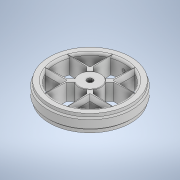
# Autodesk Inventor part: custom_wheel_v6
Saved by Autodesk Inventor 2022 (Build 260153000, 153)
## iProperties
Created: 2023-01-27
Part Number: custom_wheel_v6
Material: Generic
Document SubType Name: Modeling
Designer: user
Density: 1 g/cm^3
Appearance: Default
Author: user
Autodesk Inventor part; units mm, degrees
ref_plane "YZ Plane" through (0, 0, 0) normal (1, 0, 0) x (0, 1, 0)
ref_plane "XZ Plane" through (0, 0, 0) normal (0, 1, 0) x (-1, 0, 0)
ref_plane "XY Plane" through (0, 0, 0) normal (0, 0, 1) x (1, 0, 0)
sketch "Sketch1" plane through (0, 0, 0) normal (0, 1, 0) x (-1, 0, 0)
  circle A0 centre (0, 0) radius 37.5
  circle A1 centre (0, 0) radius 30
  circle A2 centre (0, 0) radius 10
  circle A3 centre (0, 0) radius 2.6
  dimension "d0" = 75
  dimension "d1" = 60
  dimension "d2" = 20
  dimension "d3" = 5.2
  constraints: 4 centre point, 4 coincident
  measures "d0" diameter of A0
  measures "d1" diameter of A1
  measures "d2" diameter of A2
  measures "d3" diameter of A3
extrude "Extrusion1" add sketch "Sketch1" along normal blind 15
sketch "Sketch2" plane through (0, 15, 0) normal (0, 1, 0) x (1, 0, 0)
  line L0 (0, 2.35) -> (1.1124, 2.35)
  circle A0 centre (0, 0) radius 2.6 projected
  line L1 (0, 2.35) -> (-1.1124, 2.35)
  constraints: 4 end point, 2 horizontal, 2 point on circle
extrude "Extrusion2" add sketch "Sketch2" against normal blind 15 contours L1 A0 L0 picked at (-0.5608, 2.4122)
sketch "Sketch3" plane through (-1.1124, 15, -2.35) normal (0, 0, 1) x (1, 0, 0)
  line L0 (2.2249, 0) -> (2.2249, -15) projected
  line L1 (2.2249, 0) -> (2.2249, -15)
  line L2 (11.1124, -15) -> (-8.8876, -15) projected
  line L3 (-1.4876, 0) -> (-1.4876, -15) projected
  line L4 (-1.4876, 0) -> (-1.4876, -15)
  line L5 (0, 0) -> (2.2249, 0) projected
  line L6 (1.1124, 0) -> (1.1124, -15)
  line L7 (-1.4876, -15) -> (3.7124, -15) projected
  circle A0 centre (1.1124, -7.5) radius 1.4
  point P0 (0, -15)
  point P1 (1.1124, -6.1)
  point P2 (1.1124, -8.9)
  point P3 (2.2249, -6.65)
  point P4 (2.2249, -8.35)
  dimension "d8" = 2.8
  constraints: 6 end point, 3 point on line, 2 midpoint, 1 centre point, 1 perpendicular, 1 vertical
  measures "d8" diameter of A0
extrude "Extrusion3" cut sketch "Sketch3" against normal blind 85 contours A0 L0 | L0 A0 L6 | L6 A0
sketch "Sketch5" plane through (0, 15, 0) normal (0, 1, 0) x (1, 0, 0)
  circle A0 centre (0, 0) radius 36.25
  arc A1 (-1.1124, 2.35) -> (1.1124, 2.35) centre (0, 0) ccw projected
  circle A2 centre (0, 0) radius 37.5
  dimension "d17" = 72.5
  constraints: 2 centre point, 2 coincident
  measures "d17" diameter of A0
extrude "Extrusion5" cut sketch "Sketch5" against normal blind 2.75
sketch "Sketch6" plane through (0, 0, 0) normal (0, -1, 0) x (1, 0, 0)
  circle A0 centre (0, 0) radius 37.5
  circle A1 centre (0, 0) radius 36.25
  dimension "d20" = 72.5
  constraints: 2 centre point, 2 coincident
  measures "d20" diameter of A1
extrude "Extrusion6" cut sketch "Sketch6" against normal blind 2.75
chamfer "Chamfer1" distance 1.25 angle 45 2 edges at (37.5, 12.25, 0) (37.5, 2.75, 0)
fillet "Fillet1" radius 0.4125 2 edges at (10, 0, 0) (10, 15, 0)
sketch "Sketch8" plane through (0, 15, 0) normal (0, 1, 0) x (1, 0, 0)
  line L0 (0, 0) -> (7.0711, 7.0711)
  circle A0 centre (0, 0) radius 10 projected
  line L1 (0, 0) -> (10, 0) construction
  line L2 (6.1527, 6.1527) -> (4.7385, 7.5669)
  line L3 (4.7385, 7.5669) -> (7.5669, 4.7385)
  line L4 (7.5669, 4.7385) -> (14.638, 11.8096)
  line L5 (14.638, 11.8096) -> (11.8096, 14.638)
  line L6 (11.8096, 14.638) -> (4.7385, 7.5669)
  line L7 (13.2238, 13.2238) -> (13.2238, 29.2831)
  line L8 (13.2238, 29.2831) -> (10, 30)
  line L9 (10, 30) -> (8.9811, 11.8096)
  line L10 (13.2238, 13.2238) -> (6.1527, 6.1527)
  line L11 (13.2238, 13.2238) -> (29.2831, 13.2238)
  line L12 (29.2831, 13.2238) -> (30, 10)
  line L13 (30, 10) -> (11.8096, 8.9811)
  line L14 (-13.2238, 13.2238) -> (-29.2831, 13.2238)
  line L15 (-30, 10) -> (-11.8096, 8.9811)
  line L16 (-29.2831, 13.2238) -> (-30, 10)
  line L17 (-4.7385, 7.5669) -> (-11.8096, 14.638)
  line L18 (-6.1527, 6.1527) -> (-7.5669, 4.7385)
  line L19 (-7.5669, 4.7385) -> (-4.7385, 7.5669)
  line L20 (-14.638, 11.8096) -> (-7.5669, 4.7385)
  line L21 (-13.2238, 13.2238) -> (-13.2238, 29.2831)
  line L22 (-10, 30) -> (-8.9811, 11.8096)
  line L23 (-13.2238, 29.2831) -> (-10, 30)
  line L24 (-11.8096, 14.638) -> (-14.638, 11.8096)
  line L25 (-13.2238, -13.2238) -> (-13.2238, -29.2831)
  line L26 (-10, -30) -> (-8.9811, -11.8096)
  line L27 (-13.2238, -29.2831) -> (-10, -30)
  line L28 (-7.5669, -4.7385) -> (-14.638, -11.8096)
  line L29 (-6.1527, -6.1527) -> (-4.7385, -7.5669)
  line L30 (-4.7385, -7.5669) -> (-7.5669, -4.7385)
  line L31 (-11.8096, -14.638) -> (-4.7385, -7.5669)
  line L32 (-13.2238, -13.2238) -> (-29.2831, -13.2238)
  line L33 (-30, -10) -> (-11.8096, -8.9811)
  line L34 (-29.2831, -13.2238) -> (-30, -10)
  line L35 (-14.638, -11.8096) -> (-11.8096, -14.638)
  line L36 (13.2238, -13.2238) -> (29.2831, -13.2238)
  line L37 (30, -10) -> (11.8096, -8.9811)
  line L38 (29.2831, -13.2238) -> (30, -10)
  line L39 (4.7385, -7.5669) -> (11.8096, -14.638)
  line L40 (6.1527, -6.1527) -> (7.5669, -4.7385)
  line L41 (7.5669, -4.7385) -> (4.7385, -7.5669)
  line L42 (14.638, -11.8096) -> (7.5669, -4.7385)
  line L43 (13.2238, -13.2238) -> (13.2238, -29.2831)
  line L44 (10, -30) -> (8.9811, -11.8096)
  line L45 (13.2238, -29.2831) -> (10, -30)
  line L46 (11.8096, -14.638) -> (14.638, -11.8096)
  point P0 (5.514, 8.3424)
  point P1 (8.3424, 5.514)
  point P2 (8.3424, -5.514)
  point P3 (5.514, -8.3424)
  point P4 (-8.3424, 5.514)
  point P5 (-5.514, 8.3424)
  dimension "d36" = 45
  dimension "d37" = 2
  dimension "d38" = 4
  dimension "d39" = 10
  dimension "d40" = 4
  dimension "d43" = 360
  constraints: 94 end point, 9 point on line, 3 perpendicular, 3 symmetric about line, 1 equal length, 1 horizontal, 1 midpoint, 1 vertical, 95 other
  measures "d36" angle of L1 L0
  measures "d37" distance of L2.start L2.end
  measures "d38" distance of L2.end L3.end
  measures "d39" distance of L3.end L4.end
  measures "d40" distance of L4.end L5.end
extrude "Extrusion8" add sketch "Sketch8" against normal blind 15 contours L10 L5 L4 A0 | A0 L6 L5 L10 | L11 L12 L13 L4 L5 | L5 L6 L9 L8 L7 | A0 L20 L24 L17 | L42 L46 L39 A0 | L17 L24 L21 L23 L22 | L37 L38 L36 L46 L42 | L28 L30 L29 L31 A0 | A0 L31 L35 L28 | L15 L16 L14 L24 L20 | L39 L46 L43 L45 L44 | L28 L35 L32 L34 L33 | L26 L27 L25 L35 L31
chamfer "Chamfer3" distance 3 angle 45 8 edges at (13.2238, 15, -20.076) (20.076, 15, -13.2238) (-20.076, 15, -13.2238) (-13.2238, 15, -20.076) (-20.076, 15, 13.2238) (-13.2238, 15, 20.076) (13.2238, 15, 20.076) (20.076, 15, 13.2238)
fillet "Fillet2" radius 2 12 edges at (11.7411, 15, -27.607) (27.607, 15, -11.7411) (30, 15, 0) (0, 15, -30) (-27.607, 15, -11.7411) (-11.7411, 15, -27.607) (-30, 15, 0) (-27.607, 15, 11.7411) (-11.7411, 15, 27.607) (0, 15, 30) (11.7411, 15, 27.607) (27.607, 15, 11.7411)
chamfer "Chamfer4" distance 2 angle 45 1 edges at (-1.4, 7.4985, -9.9015)
sketch "Sketch9" plane through (0, 0, 0) normal (0, -1, 0) x (1, 0, 0)
  line L0 (-1.1124, -2.35) -> (1.1124, -2.35) projected
  line L1 (0, -2.35) -> (0, -7.43)
  line L2 (0, -7.43) -> (0, -4.89)
  line L3 (0, -7.43) -> (-2.7, -7.43)
  line L4 (-2.7, -7.43) -> (2.7, -7.43)
  line L5 (2.7, -7.43) -> (2.7, -4.89)
  line L6 (2.7, -4.89) -> (-2.7, -4.89)
  line L7 (-2.7, -4.89) -> (-2.7, -7.43)
  point P0 (0, 0)
  dimension "d54" = 5.08
  dimension "d55" = 2.54
  dimension "d56" = 2.7
  dimension "d57" = 5.4
  constraints: 14 end point, 3 perpendicular, 2 midpoint, 1 horizontal, 1 point on line, 1 vertical
  measures "d54" distance of L1.start L1.end
  measures "d55" distance of L1.end L2.end
  measures "d56" distance of L1.end L3.end
  measures "d57" distance of L3.end L4.end
extrude "Extrusion9" cut sketch "Sketch9" against normal blind 13
body "Solid1"
